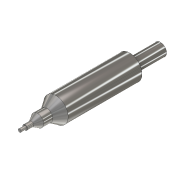
# Autodesk Inventor part: Part4
Saved by Autodesk Inventor 2017 (Build 210142000, 142)
## iProperties
Created: 2017-09-12
Part Number: Part4
Material: Nickel-Copper Alloy 400
Document SubType Name: Modeling
Designer: Amer Mohia
Density: 8.83 g/cm^3
Appearance: Chrome - Polished
Author: Amer Mohia
Autodesk Inventor part; units mm, degrees
ref_plane "YZ Plane" through (0, 0, 0) normal (1, 0, 0) x (0, 1, 0)
ref_plane "XZ Plane" through (0, 0, 0) normal (0, 1, 0) x (-1, 0, 0)
ref_plane "XY Plane" through (0, 0, 0) normal (0, 0, 1) x (1, 0, 0)
sketch "Sketch1" plane through (0, 0, 0) normal (0, 0, 1) x (1, 0, 0)
  line L0 (4.6821, 7.6658) -> (4.6821, 2.6658)
  line L1 (4.6821, 2.6658) -> (5.6821, 2.6658)
  line L2 (5.6821, 2.6658) -> (5.6821, -9.3342)
  line L3 (5.6821, -9.3342) -> (4.6821, -10.8342)
  line L4 (4.6821, -10.8342) -> (4.6821, -12.3342)
  line L5 (4.0821, -13.3342) -> (4.0821, -14.3342)
  line L6 (4.6821, -12.3342) -> (4.0821, -13.3342)
  line L7 (3.9321, -14.3342) -> (3.9321, -15.219)
  line L8 (3.6821, 7.6658) -> (3.6821, -15.2399)
  line L9 (4.0821, -14.3342) -> (3.9321, -14.3342)
  arc A0 (3.6821, -15.2399) -> (3.9321, -15.219) centre (3.7576, -14.6374) ccw
  line L10 (4.6821, 7.6658) -> (3.6821, 7.6658)
  point P0 (0, 0)
  dimension "d7" = 5
  dimension "d10" = 12
  dimension "d14" = 1
  dimension "d17" = 1.5
  dimension "d18" = 3
  dimension "d19" = 1
  dimension "d21" = 0.5
  dimension "d22" = 0.8
  dimension "d23" = 2
  dimension "d24" = 4
  dimension "d25" = 2
  constraints: 22 end point, 5 vertical, 3 perpendicular, 2 point on circle, 1 centre point, 1 horizontal
  measures "d7" distance of L0.start L0.end
  measures "d10" distance of L1.end L2.end
  measures "d14" vertical distance of L4.end L5.start
  measures "d17" vertical distance of L2.end L3.end
  measures "d18" vertical distance of L4.end L2.end
  measures "d19" distance of L5.start L5.end
  measures "d21" diameter of L7 L8
  measures "d22" diameter of L5 L8
  measures "d23" diameter of L4 L8
  measures "d24" diameter of L2 L8
  measures "d25" diameter of L0 L8
revolve "Revolution1" add sketch "Sketch1" angle 360 about axis through (3.6821, 7.6658, 0) along (0, -1, 0)
body "Solid1"
